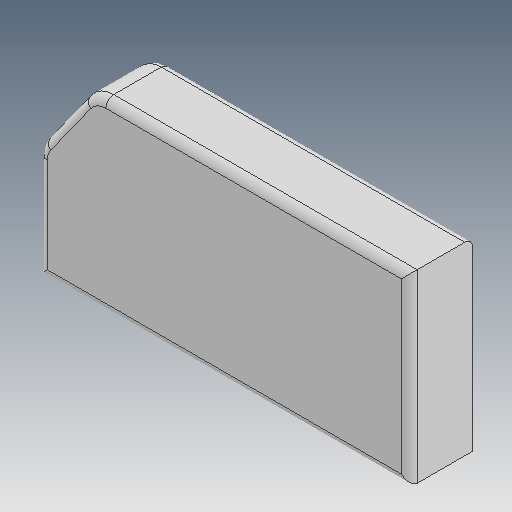
# Autodesk Inventor part: Armlehne Polsterung
Saved by Autodesk Inventor 2020 (Build 240168000, 168)
## iProperties
Created: 2022-03-11
Part Number: Armlehne Polsterung
Material: Generisch
Document SubType Name: Modeling
Designer: Mike
Density: 1 g/cm^3
Appearance: Vorgabe
Author: Mike
Autodesk Inventor part; units mm, degrees
ref_plane "YZ Plane" through (0, 0, 0) normal (1, 0, 0) x (0, 1, 0)
ref_plane "XZ Plane" through (0, 0, 0) normal (0, 1, 0) x (-1, 0, 0)
ref_plane "XY Plane" through (0, 0, 0) normal (0, 0, 1) x (1, 0, 0)
sketch "Skizze1" plane through (0, 0, 0) normal (0, 0, 1) x (1, 0, 0)
  line L0 (-171.7282, 72.7948) -> (402.5409, 72.7948)
  line L1 (402.5409, 72.7948) -> (402.5409, -277.2052)
  line L2 (402.5409, -277.2052) -> (-297.4591, -277.2052)
  line L3 (-297.4591, -277.2052) -> (-297.4591, -83.2285)
  line L4 (-212.4149, 51.8567) -> (-288.1458, -54.1666)
  arc A0 (-171.7282, 72.7948) -> (-212.4149, 51.8567) centre (-171.7282, 22.7948) ccw
  arc A1 (-288.1458, -54.1666) -> (-297.4591, -83.2285) centre (-247.4591, -83.2285) ccw
  point P0 (0, 0)
  point P1 (-297.4591, -67.2052)
  point P2 (-197.4591, 72.7948)
  dimension "d0" = 700
  dimension "d1" = 350
  dimension "d2" = 210
  dimension "d3" = 600
  dimension "d4" = 50
  constraints: 10 end point, 4 point on circle, 4 point on line, 4 tangent, 2 centre point, 2 parallel, 1 equal radius, 1 horizontal, 1 perpendicular
  measures "d0" distance of L1.end L2.end
  measures "d1" distance of L0.end L1.end
  measures "d2" distance of L2.end point (-297.459, -67.205)
  measures "d3" distance of point (-197.459, 72.795) L0.end
  measures "d4" radius of A0
extrude "Extrusion1" add sketch "Skizze1" along normal blind 120
fillet "Rundung1" radius 15 12 edges at (-194.6073, 67.2532, 120) (-250.2803, -1.1549, 120) (-295.0739, -67.9696, 120) (-297.4591, -180.2168, 120) (115.4064, 72.7948, 120) (-194.6073, 67.2532, 0) (-250.2803, -1.1549, 0) (-295.0739, -67.9696, 0) (-297.4591, -180.2168, 0) (115.4064, 72.7948, 0) (402.5409, -102.2052, 120) (52.5409, -277.2052, 120)
